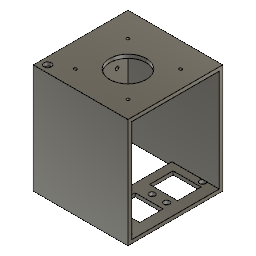
Power_3d_Project (Autodesk Fusion 360 design; units mm, degrees)
Autodesk Fusion 360 part; units mm, degrees
sketch "body_dimension" plane through (0, 0, 0) normal (0, 0, 1) x (1, 0, 0) in component "case"
  line L0 (0, 0) -> (130, 0)
  line L1 (130, 0) -> (130, 130)
  line L2 (130, 130) -> (0, 130)
  line L3 (0, 130) -> (0, 0)
  dimension "d1" = 130
  dimension "d2" = 130
  constraint horizontal L0
  constraint vertical L1
  constraint horizontal L2
  constraint vertical L3
  constraint coincident L0.start L3.end
  measures "d1" distance of L0.start L0.end
  measures "d2" distance of L0.start L2.end
extrude "Extrude2" add sketch "body_dimension" along normal blind 150 in component "case"
sketch "back" plane through (0, 0, 150) normal (0, 0, 1) x (-1, 0, 0) in component "case"
  line L0 (0, -130) -> (0, 0)
  line L1 (0, 0) -> (-130, 0)
  line L2 (-130, 0) -> (-130, -130)
  line L3 (-130, -130) -> (0, -130)
  circle A0 centre (-10, -10) radius 5
  circle A1 centre (-34, -96) radius 2
  line L4 (-130, 0) -> (-130, -130)
  line L5 (-130, -130) -> (0, -130)
  circle A2 centre (-106, -96) radius 2
  circle A3 centre (-106, -24) radius 2
  circle A4 centre (-34, -24) radius 2
  circle A5 centre (-70, -60) radius 25
  dimension "d9" = 10
  dimension "d14" = 4
  dimension "d86" = 4
  dimension "d89" = 4
  dimension "d92" = 4
  dimension "d95" = 50
  dimension "d96" = 60
  dimension "d97" = 70
  measures "d9" diameter of A0
  measures "d14" diameter of A1
  measures "d86" diameter of A2
  measures "d89" diameter of A3
  measures "d92" diameter of A4
  measures "d95" diameter of A5
  measures "d96" distance of L1 A5.centre
  measures "d97" distance of L0 A5.centre
shell "Shell1" thickness 5 removed faces 1 at (130, 43.3333, 50) in component "case"
sketch "front" plane through (0, 0, 0) normal (0, 0, 1) x (1, 0, 0) in component "case"
  line L0 (115, 83) -> (76.8, 83)
  line L1 (76.8, 83) -> (76.8, 115)
  line L2 (76.8, 115) -> (115, 115)
  line L3 (115, 115) -> (115, 83)
  line L4 (130, 0) -> (130, 130)
  line L5 (130, 130) -> (0, 130)
  line L6 (65, 68) -> (5, 68)
  line L7 (5, 68) -> (5, 125)
  line L8 (5, 125) -> (65, 125)
  line L9 (65, 125) -> (65, 68)
  line L10 (115, 31) -> (76.8, 31)
  line L11 (76.8, 31) -> (76.8, 63)
  line L12 (76.8, 63) -> (115, 63)
  line L13 (115, 63) -> (115, 31)
  line L14 (0, 0) -> (130, 0)
  circle A0 centre (120, 10) radius 4
  circle A1 centre (90, 10) radius 5
  circle A2 centre (60, 10) radius 3.5
  circle A3 centre (43.3333, 10) radius 3.5
  circle A4 centre (26.6667, 10) radius 3.5
  circle A5 centre (10, 10) radius 3.5
  circle A6 centre (60, 25) radius 3.5
  circle A7 centre (43.3333, 25) radius 3.5
  circle A8 centre (26.6667, 25) radius 3.5
  circle A9 centre (10, 25) radius 3.5
  circle A10 centre (60, 40) radius 3.5
  circle A11 centre (43.3333, 40) radius 3.5
  circle A12 centre (26.6667, 40) radius 3.5
  circle A13 centre (10, 40) radius 3.5
  circle A14 centre (60, 55) radius 3.5
  circle A15 centre (43.3333, 55) radius 3.5
  circle A16 centre (26.6667, 55) radius 3.5
  circle A17 centre (10, 55) radius 3.5
  circle A18 centre (110, 10) radius 2.5
  circle A19 centre (51.6667, 17.5) radius 2.5
  circle A20 centre (51.6667, 47.5) radius 2.5
  circle A21 centre (110, 73) radius 4
  circle A22 centre (90, 73) radius 4
  circle A23 centre (110, 122) radius 4
  line L15 (0, 0) -> (0, 130)
  line L16 (0, 130) -> (130, 130)
  line L17 (130, 130) -> (130, 0)
  line L18 (130, 0) -> (0, 0)
  dimension "d20" = 38.2
  dimension "d21" = 32
  dimension "d22" = 15
  dimension "d23" = 15
  dimension "d24" = 60
  dimension "d25" = 57
  dimension "d26" = 5
  dimension "d27" = 65
  dimension "d28" = 38.2
  dimension "d29" = 32
  dimension "d30" = 15
  dimension "d31" = 20
  dimension "d36" = 8
  dimension "d37" = 10
  dimension "d38" = 10
  dimension "d39" = 10
  dimension "d40" = 10
  dimension "d41" = 30
  dimension "d42" = 7
  dimension "d43" = 10
  dimension "d44" = 70
  dimension "d47" = 50
  dimension "d48" = -45
  dimension "d49" = 16.6667
  dimension "d50" = 16.6667
  dimension "d51" = 16.6667
  dimension "d52" = 15
  dimension "d53" = 15
  dimension "d54" = 15
  dimension "d56" = 5
  dimension "d57" = 20
  dimension "d58" = 10
  dimension "d59" = 5
  dimension "d72" = 5
  dimension "d75" = 8
  dimension "d76" = 73
  dimension "d77" = 20
  dimension "d78" = 8
  dimension "d79" = 73
  dimension "d80" = 40
  dimension "d81" = 8
  dimension "d82" = 20
  dimension "d83" = 8
  constraint horizontal L0
  constraint vertical L1
  constraint horizontal L2
  constraint vertical L3
  constraint horizontal L6
  constraint vertical L7
  constraint horizontal L8
  constraint vertical L9
  constraint horizontal L10
  constraint vertical L11
  constraint horizontal L12
  constraint vertical L13
  measures "d20" distance of L0.start L0.end
  measures "d21" distance of L0.start L2.end
  measures "d22" distance of L2.end L4
  measures "d23" distance of L2.end L5
  measures "d24" distance of L6.start L6.end
  measures "d25" distance of L6.start L8.end
  measures "d26" distance of L5 L8.end
  measures "d27" distance of L4 L8.end
  measures "d28" distance of L10.start L10.end
  measures "d29" distance of L10.start L12.end
  measures "d30" distance of L4 L12.end
  measures "d31" distance of L0.start L12.end
  measures "d36" diameter of A0
  measures "d37" distance of L4 A0.centre
  measures "d38" distance of L14 A0.centre
  measures "d39" diameter of A1
  measures "d40" distance of L14 A1.centre
  measures "d41" distance of A0.centre A1.centre
  measures "d42" diameter of A2
  measures "d43" distance of L14 A2.centre
  measures "d44" distance of L4 A2.centre
  measures "d49" distance of A2.centre A3.centre
  measures "d50" distance of A3.centre A4.centre
  measures "d51" distance of A4.centre A5.centre
  measures "d52" distance of A2.centre A6.centre
  measures "d53" distance of A6.centre A10.centre
  measures "d54" distance of A10.centre A14.centre
  measures "d56" diameter of A18
  measures "d57" distance of L4 A18.centre
  measures "d58" distance of L14 A18.centre
  measures "d59" diameter of A19
  measures "d72" diameter of A20
  measures "d75" diameter of A21
  measures "d76" distance of L14 A21.centre
  measures "d77" distance of L4 A21.centre
  measures "d78" diameter of A22
  measures "d79" distance of L14 A22.centre
  measures "d80" distance of L4 A22.centre
  measures "d81" diameter of A23
  measures "d82" distance of L4 A23.centre
  measures "d83" distance of L5 A23.centre
extrude "Extrude3" cut sketch "back" against normal blind 5 contours A0 in component "case"
extrude "Extrude4" cut sketch "front" along normal blind 5 contours L10 L11 L12 L13 in component "case"
extrude "Extrude5" cut sketch "front" along normal blind 5 contours L0 L1 L2 L3 in component "case"
extrude "Extrude6" cut sketch "front" along normal blind 5 contours L6 L7 L8 L9 in component "case"
extrude "Extrude7" cut sketch "front" along normal blind 5 contours A0 | A1 | A2 | A3 | A4 | A6 | A7 | A8 | A10 | A11 | A12 | A14 | A15 | A16 | A18 in component "case"
extrude "Extrude8" cut sketch "front" along normal blind 5 contours A4 | A5 | A8 | A9 | A12 | A13 | A16 | A17 in component "case"
extrude "Extrude9" cut sketch "front" along normal blind 5 contours A19 | A20 in component "case"
extrude "Extrude10" cut sketch "front" along normal blind 5 contours A21 | A22 | A23 in component "case"
extrude "Extrude11" cut sketch "back" against normal blind 5 contours A5 in component "case"
extrude "Extrude12" cut sketch "back" against normal blind 5 contours A1 | A2 | A3 | A4 in component "case"
sketch "bottom" plane through (0, 0, 0) normal (-1, 0, 0) x (0, -1, 0) in component "case"
  line L0 (-130, 0) -> (0, 0)
  line L1 (0, 0) -> (0, 150)
  line L2 (0, 150) -> (-130, 150)
  line L3 (-130, 150) -> (-130, 0)
  circle A0 centre (-20, 20) radius 2.5
  line L4 (-130, 0) -> (0, 0)
  circle A1 centre (-50, 20) radius 2.5
  circle A2 centre (-80, 20) radius 2.5
  circle A3 centre (-110, 20) radius 2.5
  circle A4 centre (-20, 56.6667) radius 2.5
  circle A5 centre (-50, 56.6667) radius 2.5
  circle A6 centre (-80, 56.6667) radius 2.5
  circle A7 centre (-110, 56.6667) radius 2.5
  circle A8 centre (-20, 93.3333) radius 2.5
  circle A9 centre (-50, 93.3333) radius 2.5
  circle A10 centre (-80, 93.3333) radius 2.5
  circle A11 centre (-110, 93.3333) radius 2.5
  circle A12 centre (-20, 130) radius 2.5
  circle A13 centre (-50, 130) radius 2.5
  circle A14 centre (-80, 130) radius 2.5
  circle A15 centre (-110, 130) radius 2.5
  dimension "d102" = 5
  dimension "d103" = 20
  dimension "d104" = 20
  dimension "d109" = -90
  dimension "d110" = 110
  measures "d102" diameter of A0
  measures "d103" distance of A0.centre L4
  measures "d104" distance of L1 A0.centre
extrude "Extrude13" cut sketch "bottom" against normal blind 5 contours A0 in component "case"
extrude "Extrude15" cut sketch "bottom" against normal blind 5 contours A1 | A2 | A3 | A4 | A5 | A6 | A7 | A8 | A9 | A10 in component "case"
extrude "Extrude16" cut sketch "bottom" against normal blind 5 contours A11 in component "case"
extrude "Extrude17" cut sketch "bottom" against normal blind 5 contours A12 | A13 | A14 | A15 in component "case"
extrude "Extrude14" [suppressed] in component "case"
extrude "Extrude1" [rolled back] along distance 50 taper angle 0 in component "case"
sketch "Sketch2" plane through (0, 0, 0) normal (0, -1, 0) x (1, 0, 0) in component "case"
  line L0 (0, 0) -> (100, 0)
  line L1 (100, 0) -> (100, 50)
  line L2 (100, 50) -> (0, 50)
  line L3 (0, 50) -> (0, 0)
component "case" placed x (1, 0, 0) y (0, 1, 0) z (0, 0, 1) at (0, 0, 0)
named bodies: "z_height"
